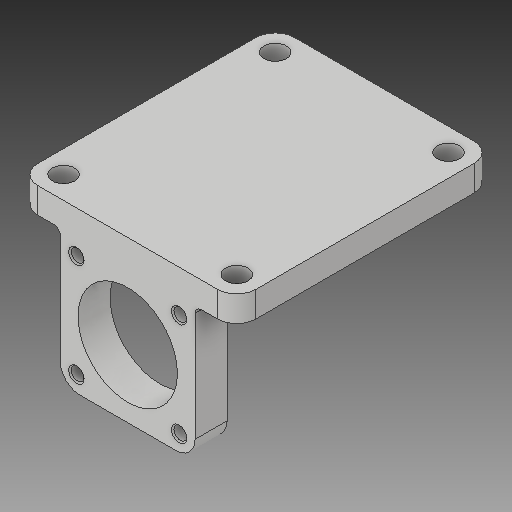
# Autodesk Inventor part: Nema8_holder
Saved by Autodesk Inventor 2019 (Build 230136000, 136)
## iProperties
Created: 2021-10-06
Part Number: Nema8_holder
Material: Generic
Document SubType Name: Modeling
Designer: Pokick
Density: 1 g/cm^3
Appearance: Default
Author: Pokick
Autodesk Inventor part; units mm, degrees
ref_plane "YZ Plane" through (0, 0, 0) normal (1, 0, 0) x (0, 1, 0)
ref_plane "XZ Plane" through (0, 0, 0) normal (0, 1, 0) x (-1, 0, 0)
ref_plane "XY Plane" through (0, 0, 0) normal (0, 0, 1) x (1, 0, 0)
sketch "Sketch1" plane through (0, 0, 0) normal (0, 0, 1) x (1, 0, 0)
  line L0 (8, -8) -> (-8, -8) construction
  line L1 (-8, -8) -> (-8, 8) construction
  line L2 (-8, 8) -> (8, 8) construction
  line L3 (8, 8) -> (8, -8) construction
  line L4 (8, -8) -> (-8, 8) construction
  line L5 (-8, -8) -> (8, 8) construction
  circle A0 centre (0, 0) radius 7.75
  line L6 (10.5, -10.5) -> (-10.5, -10.5)
  line L7 (-10.5, -10.5) -> (-10.5, 10.5)
  line L8 (-10.5, 10.5) -> (10.5, 10.5)
  line L9 (10.5, 10.5) -> (10.5, -10.5)
  line L10 (10.5, -10.5) -> (-10.5, 10.5) construction
  line L11 (-10.5, -10.5) -> (10.5, 10.5) construction
  circle A1 centre (-8, -8) radius 1
  circle A2 centre (8, -8) radius 1
  circle A3 centre (8, 8) radius 1
  circle A4 centre (-8, 8) radius 1
  dimension "d0" = 16
  dimension "d1" = 16
  dimension "d2" = 15.5
  dimension "d3" = 21
  dimension "d4" = 21
  dimension "d5" = 2
  dimension "d8" = 360
  constraints: 24 end point, 5 centre point, 4 midpoint, 4 parallel, 2 coincident, 2 horizontal, 2 perpendicular, 9 other
  measures "d0" distance of L1.end L2.end
  measures "d1" distance of L0.end L1.end
  measures "d2" diameter of A0
  measures "d3" distance of L7.end L8.end
  measures "d4" distance of L6.end L7.end
  measures "d5" diameter of A1
extrude "Extrusion1" add sketch "Sketch1" along normal blind 5
sketch "Sketch2" plane through (-10.5, 10.5, 0) normal (0, 1, 0) x (1, 0, 0)
  line L0 (10.5, 0) -> (-6.5, 0) construction
  line L1 (-6.5, 0) -> (-6.5, -5) construction
  line L2 (-6.5, -5) -> (10.5, -5) construction
  line L3 (10.5, -5) -> (10.5, 0) construction
  line L4 (-6.5, -5) -> (27.5, -5)
  line L5 (27.5, -5) -> (27.5, 35)
  line L6 (27.5, 35) -> (-6.5, 35)
  line L7 (-6.5, 35) -> (-6.5, -5)
  line L8 (27.5, 35) -> (-6.5, -5) construction
  line L9 (-6.5, 35) -> (27.5, -5) construction
  line L10 (-3, 31.5) -> (24, 31.5) construction
  line L11 (24, 31.5) -> (24, -1.5) construction
  line L12 (24, -1.5) -> (-3, -1.5) construction
  line L13 (-3, -1.5) -> (-3, 31.5) construction
  line L14 (-3, 31.5) -> (24, -1.5) construction
  line L15 (24, 31.5) -> (-3, -1.5) construction
  circle A0 centre (24, -1.5) radius 1.75
  circle A1 centre (-3, -1.5) radius 1.75
  circle A2 centre (-3, 31.5) radius 1.75
  circle A3 centre (24, 31.5) radius 1.75
  point P0 (10.5, 15)
  dimension "d12" = 17
  dimension "d13" = 5
  dimension "d14" = 34
  dimension "d15" = 40
  dimension "d16" = 27
  dimension "d17" = 33
  dimension "d18" = 3.5
  dimension "d19" = 3.5
  dimension "d20" = 3.5
  dimension "d21" = 3.5
  constraints: 32 end point, 6 parallel, 4 centre point, 4 coincident, 3 horizontal, 3 midpoint, 3 perpendicular
  measures "d12" distance of L2.end L1.end
  measures "d13" distance of L1.end L0.end
  measures "d14" distance of L6.end L5.end
  measures "d15" distance of L5.end L4.end
  measures "d16" distance of L11.end L12.end
  measures "d17" distance of L10.end L11.end
  measures "d18" diameter of A0
  measures "d19" diameter of A1
  measures "d20" diameter of A2
  measures "d21" diameter of A3
extrude "Extrusion2" add sketch "Sketch2" along normal blind 4
fillet "Fillet2" radius 3 2 edges at (-10.5, -10.5, 2.5) (10.5, -10.5, 2.5)
fillet "Fillet3" radius 3 4 edges at (17, 12.5, 5) (-17, 12.5, 5) (17, 12.5, -35) (-17, 12.5, -35)
fillet "Fillet4" radius 0.4 1 edges at (0, 10.5, 0)
chamfer "Chamfer1" distance 0.2 angle 45 4 edges at (11.75, 10.5, 1.5) (11.75, 10.5, -31.5) (-15.25, 10.5, -31.5) (-15.25, 10.5, 1.5)
fillet "Fillet5" radius 1 4 edges at (10.5, 10.5, -0.2) (10.5, 10.5, 2.5) (-10.5, 10.5, -0.2) (-10.5, 10.5, 2.5)
chamfer "Chamfer2" distance 0.2 angle 45 4 edges at (7, -8, 5) (-9, -8, 5) (-9, 8, 5) (7, 8, 5)
body "Solid1"
